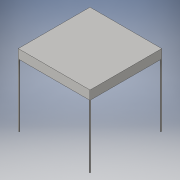
# Autodesk Inventor part: Pit
Saved by Autodesk Inventor 2016 SP2 (Build 200236200, 236)
## iProperties
Created: 2018-01-20
Part Number: Pit
Material: Generic
Document SubType Name: Modeling
Designer: CAD
Density: 1 g/cm^3
Appearance: Default
Author: CAD
Autodesk Inventor part; units mm, degrees
ref_plane "YZ Plane" through (0, 0, 0) normal (1, 0, 0) x (0, 1, 0)
ref_plane "XZ Plane" through (0, 0, 0) normal (0, 1, 0) x (-1, 0, 0)
ref_plane "XY Plane" through (0, 0, 0) normal (0, 0, 1) x (1, 0, 0)
sketch "Sketch1" plane through (0, 0, 0) normal (0, 0, 1) x (1, 0, 0)
  line L0 (0, 0) -> (0, 2438.4)
  line L1 (0, 2438.4) -> (2438.4, 2438.4)
  line L2 (2409.825, 2133.6) -> (28.575, 2133.6)
  line L3 (2438.4, 2438.4) -> (2438.4, 0)
  line L4 (2409.825, 0) -> (2409.825, 2133.6)
  line L5 (28.575, 2133.6) -> (28.575, 0)
  line L6 (0, 0) -> (28.575, 0)
  line L7 (2409.825, 0) -> (2438.4, 0)
  dimension "d0" = 0
  dimension "d1" = 2438.4
  dimension "d3" = 2438.4
  dimension "d4" = 304.8
  dimension "d5" = 28.575
  dimension "d7" = 28.575
  constraints: 16 end point, 2 horizontal, 1 collinear, 1 parallel, 1 vertical
  measures "d0" horizontal distance of L0.start L0.end
  measures "d1" distance of L0.start L0.end
  measures "d3" distance of L0.end L1.end
  measures "d4" distance between parallel lines of L1 L2
  measures "d5" distance between parallel lines of L3 L4
  measures "d7" distance between parallel lines of L0 L5
extrude "Extrusion1" add sketch "Sketch1" along normal blind 2438.4
sketch "Sketch2" plane through (2438.4, 0, 0) normal (1, 0, 0) x (0, 0, -1)
  line L0 (0, 2438.4) -> (-2438.4, 2438.4) projected
  line L1 (-2438.4, 0) -> (-2438.4, 2438.4) projected
  line L2 (0, 2438.4) -> (0, 0) projected
  line L3 (-2409.825, 0) -> (-2409.825, 2133.6)
  line L4 (-28.575, 2133.6) -> (-28.575, 0)
  line L5 (-2409.825, 2133.6) -> (-28.575, 2133.6)
  line L6 (0, 0) -> (-2438.4, 0) projected
  line L7 (-2409.825, 0) -> (-28.575, 0)
  dimension "d10" = 28.575
  dimension "d11" = 28.575
  dimension "d12" = 2133.6
  dimension "d13" = 2133.6
  dimension "d14" = 304.8
  constraints: 8 end point, 1 horizontal
  measures "d10" distance between parallel lines of L1 L3
  measures "d11" distance between parallel lines of L2 L4
  measures "d12" distance of L3.start L3.end
  measures "d13" distance of L4.start L4.end
  measures "d14" distance between parallel lines of L5 L0
extrude "Extrusion2" cut sketch "Sketch2" against normal blind 2438.4 contours L6 L3 L5 L4
sketch "Sketch3" plane through (28.575, 2133.6, 0) normal (0, -1, 0) x (1, 0, 0)
  line L0 (2381.25, 2409.825) -> (2381.25, 2438.4) projected
  line L1 (0, 2409.825) -> (0, 2438.4) projected
  line L2 (2381.25, 2409.825) -> (0, 2409.825)
  line L3 (0, 28.575) -> (-28.575, 28.575) projected
  line L4 (0, 2409.825) -> (0, 28.575)
  line L5 (0, 28.575) -> (2381.25, 28.575)
  line L6 (2381.25, 28.575) -> (2381.25, 2409.825)
  point P0 (-28.575, 0)
  constraints: 8 end point, 3 perpendicular, 1 horizontal
extrude "Extrusion3" cut sketch "Sketch3" against normal blind 276.225
sketch "Sketch4" plane through (28.575, 2133.6, 28.575) normal (0, 0, 1) x (1, 0, 0)
  line L0 (2381.25, 0) -> (2381.25, 276.225) projected
  line L1 (2381.25, 276.225) -> (0, 276.225) projected
  line L2 (0, 0) -> (0, 276.225) projected
  line L3 (-28.575, 304.8) -> (2409.825, 304.8) projected
  line L4 (0, 276.225) -> (2381.25, 276.225) projected
  line L5 (1190.625, 276.225) -> (1190.625, 0)
  line L6 (0, 276.225) -> (550.3563, 148.5423)
  line L7 (595.3125, 138.1125) -> (1190.625, 0)
  line L8 (0, 20.8597) -> (550.3563, 148.5423)
  line L9 (595.3125, 158.9722) -> (1100.7126, 276.225)
  line L10 (89.9124, 276.225) -> (595.3125, 158.9722)
  line L11 (640.2687, 148.5423) -> (1190.625, 20.8597)
  line L12 (0, 0) -> (595.3125, 138.1125)
  line L13 (640.2687, 148.5423) -> (1190.625, 276.225)
  line L14 (2381.25, 0) -> (1785.9375, 138.1125)
  line L15 (1740.9813, 148.5423) -> (1190.625, 276.225)
  line L16 (2291.3376, 276.225) -> (1785.9375, 158.9722)
  line L17 (1740.9813, 148.5423) -> (1190.625, 20.8597)
  line L18 (2381.25, 20.8597) -> (1830.8937, 148.5423)
  line L19 (1785.9375, 158.9722) -> (1280.5374, 276.225)
  line L20 (2381.25, 276.225) -> (1830.8937, 148.5423)
  line L21 (1785.9375, 138.1125) -> (1190.625, 0)
  point P0 (-28.575, -2133.6)
  point P1 (2385.8423, 19.7943)
  point P2 (1195.2173, 296.0193)
  point P3 (2376.6577, 296.0193)
  point P4 (-4.5923, 19.7943)
  point P5 (1186.0327, 296.0193)
  point P6 (4.5923, 296.0193)
  dimension "d26" = 606.4093
  dimension "d29" = 518.8231
  dimension "d31" = 564.9734
  dimension "d34" = 611.1236
  dimension "d35" = 611.1236
  dimension "d36" = 569.6876
  dimension "d37" = 564.9734
  dimension "d38" = 564.9734
  dimension "d39" = 89.9124
  dimension "d40" = 1010.8001
  dimension "d41" = 1010.8001
  dimension "d42" = 564.9734
  dimension "d43" = 564.9734
  constraints: 34 end point, 7 equal length, 7 point on line, 4 parallel, 3 symmetric about line, 1 midpoint, 1 perpendicular
  measures "d26" distance of point (4.592, 296.019) L9.start
  measures "d29" distance of L9.start L9.end
  measures "d31" distance of L11.start L5.start
  measures "d34" distance of L7.start L5.end
  measures "d35" distance of L2.start L7.start
  measures "d36" distance of point (-4.592, 19.794) L6.end
  measures "d37" distance of L1.end L6.end
  measures "d38" distance of L11.start L11.end
  measures "d39" distance of L11.start L6.end
  measures "d40" distance of L9.end L10.start
  measures "d41" distance of L16.start L19.end
  measures "d42" distance of L8.start L6.end
  measures "d43" distance of L18.start L18.end
extrude "Extrusion4" add sketch "Sketch4" along normal blind 20.32 contours L14 L21 L5 L17 L15 L1 L19 L16 L20 L18 L0 | L7 L12 L2 L8 L6 L1 L10 L9 L13 L11 L5
sketch "Sketch6" plane through (28.575, 2133.6, 2409.825) normal (1, 0, 0) x (0, 0, -1)
  line L0 (2360.93, 276.225) -> (0, 276.225) projected
  line L1 (1180.465, 276.225) -> (1180.465, 0)
  line L2 (2381.25, 276.225) -> (2360.93, 276.225) projected
  line L3 (2381.25, 276.225) -> (2381.25, 0)
  line L4 (1180.465, 276.225) -> (1717.1258, 152.7732)
  line L5 (1780.8575, 138.1125) -> (2381.25, 0)
  line L6 (2253.7866, 276.225) -> (1780.8575, 167.4338)
  line L7 (1717.1258, 152.7732) -> (1180.465, 29.3213)
  line L8 (2381.25, 29.3213) -> (1844.5892, 152.7732)
  line L9 (1780.8575, 167.4338) -> (1307.9284, 276.225)
  line L10 (1180.465, 0) -> (1780.8575, 138.1125)
  line L11 (1844.5892, 152.7732) -> (2381.25, 276.225)
  line L12 (-20.32, 29.3213) -> (-20.32, 0)
  line L13 (1180.465, 276.225) -> (643.8042, 152.7732)
  line L14 (580.0725, 138.1125) -> (0, 4.6744)
  line L15 (107.1434, 276.225) -> (580.0725, 167.4338)
  line L16 (643.8042, 152.7732) -> (1180.465, 29.3213)
  line L17 (0, 33.9957) -> (516.3408, 152.7732)
  line L18 (580.0725, 167.4338) -> (1053.0016, 276.225)
  line L19 (1180.465, 0) -> (580.0725, 138.1125)
  line L20 (516.3408, 152.7732) -> (0, 276.225)
  line L21 (0, 33.9957) -> (0, 4.6744)
  line L22 (0, 0) -> (0, 276.225) projected
  line L23 (2253.7866, 276.225) -> (2381.25, 276.225)
  line L24 (107.1434, 276.225) -> (0, 276.225)
  line L25 (1053.0016, 276.225) -> (1180.465, 276.225)
  line L26 (2253.7866, 276.225) -> (2381.25, 276.225)
  line L27 (2409.825, 304.8) -> (-28.575, 304.8) projected
  line L28 (2381.25, 0) -> (2360.93, 0) projected
  line L29 (2381.25, 0) -> (2381.25, 29.3213)
  line L30 (2381.25, 20.8597) -> (2381.25, 148.5423) projected
  point P0 (2409.825, -2133.6)
  point P1 (-20.32, 276.225)
  dimension "d68" = 28.575
  dimension "d69" = 28.575
  dimension "d70" = 28.575
  dimension "d71" = 28.575
  dimension "d73" = 616.0732
  dimension "d75" = 485.2808
  dimension "d76" = 485.2808
  dimension "d77" = 25.91
  dimension "d79" = 276.225
  dimension "d80" = 167.045
  dimension "d81" = 167.045
  dimension "d82" = 20.32
  dimension "d83" = 276.225
  constraints: 50 end point, 8 point on line, 7 symmetric about line, 3 parallel, 2 perpendicular, 1 collinear, 1 midpoint
  measures "d68" distance between parallel lines of L9 L4
  measures "d69" distance between parallel lines of L5 L8
  measures "d70" distance between parallel lines of L6 L11
  measures "d71" distance between parallel lines of L10 L7
  measures "d73" distance of L1.end L5.start
  measures "d75" distance of L6.end L9.end
  measures "d76" distance of L6.start L6.end
  measures "d77" angle of L11 L8
  measures "d79" distance of L1.start L1.end
  measures "d80" angle of L2 L14
  measures "d81" angle of L2 L17
  measures "d82" distance between parallel lines of L12 L22
  measures "d83" distance from line of L12.end L0
extrude "Extrusion5" add sketch "Sketch6" along normal blind 20.32 contours L2 L11 L8 L3 L5 L10 L1 L7 L4 L0 L9 L6 | L13 L16 L1 L19 L14 L21 L17 L20 L0 L15 L18
sketch "Sketch7" plane through (2409.825, 2133.6, 2409.825) normal (0, 0, -1) x (-1, 0, 0)
  line L0 (0, 276.225) -> (550.3563, 148.5423) projected
  line L1 (550.3563, 148.5423) -> (0, 20.8597) projected
  line L2 (595.3125, 138.1125) -> (1190.625, 0) projected
  line L3 (1100.7126, 276.225) -> (595.3125, 158.9722) projected
  line L4 (640.2687, 148.5423) -> (1190.625, 276.225) projected
  line L5 (1190.625, 20.8597) -> (640.2687, 148.5423) projected
  line L6 (0, 0) -> (595.3125, 138.1125) projected
  line L7 (595.3125, 158.9722) -> (89.9124, 276.225) projected
  line L8 (2409.825, 304.8) -> (-28.575, 304.8) projected
  line L9 (1190.625, 0) -> (1785.9375, 138.1125) projected
  line L10 (1190.625, 276.225) -> (1740.9813, 148.5423) projected
  line L11 (1785.9375, 158.9722) -> (1280.5374, 276.225) projected
  line L12 (1740.9813, 148.5423) -> (1190.625, 20.8597) projected
  line L13 (1785.9375, 138.1125) -> (2360.93, 4.7142) projected
  line L14 (2360.93, 25.5739) -> (1830.8937, 148.5423) projected
  line L15 (2291.3376, 276.225) -> (1785.9375, 158.9722) projected
  line L16 (2381.25, 276.225) -> (2360.93, 276.225) projected
  line L17 (1830.8937, 148.5423) -> (2381.25, 276.225)
  line L18 (0, 276.225) -> (89.9124, 276.225)
  line L19 (0, 0) -> (0, 20.8597)
  line L20 (2291.3376, 276.225) -> (2381.25, 276.225)
  line L21 (1100.7126, 276.225) -> (1280.5374, 276.225)
  line L22 (0, 0) -> (0, 20.8597)
  line L23 (595.3125, 138.1125) -> (0, 0)
  line L24 (0, 20.8597) -> (550.3563, 148.5423)
  line L25 (0, 276.225) -> (550.3563, 148.5423)
  line L26 (595.3125, 158.9722) -> (89.9124, 276.225)
  line L27 (595.3125, 158.9722) -> (1100.7126, 276.225)
  line L28 (1190.625, 276.225) -> (640.2687, 148.5423)
  line L29 (640.2687, 148.5423) -> (1190.625, 20.8597)
  line L30 (1190.625, 0) -> (595.3125, 138.1125)
  line L31 (1190.625, 0) -> (1785.9375, 138.1125)
  line L32 (1190.625, 20.8597) -> (1740.9813, 148.5423)
  line L33 (1190.625, 276.225) -> (1740.9813, 148.5423)
  line L34 (1785.9375, 158.9722) -> (1280.5374, 276.225)
  line L35 (1785.9375, 158.9722) -> (2291.3376, 276.225)
  line L36 (1830.8937, 148.5423) -> (2360.93, 25.5739)
  line L37 (2360.93, 4.6744) -> (2360.93, 25.5739)
  line L38 (2360.93, 4.6744) -> (1785.9375, 138.1125)
  point P0 (2361.1019, 271.5506)
  point P1 (2381.25, 0)
  dimension "d88" = 13.062
  dimension "d89" = 166.6875
  constraints: 44 end point, 10 collinear, 4 parallel, 1 perpendicular
  measures "d88" angle of L8 L30
  measures "d89" distance from line of L30.end L8
extrude "Extrusion6" add sketch "Sketch7" along normal blind 20.32
sketch "Sketch8" plane through (2409.825, 2154.4597, 28.575) normal (-1, 0, 0) x (0, 0, 1)
  line L0 (20.32, -16.1853) -> (600.3925, 117.2528) projected
  line L1 (536.6608, 131.9135) -> (0, 8.4616) projected
  line L2 (0, 255.3653) -> (536.6608, 131.9135) projected
  line L3 (600.3925, 146.5741) -> (127.4634, 255.3653) projected
  line L4 (1073.3216, 255.3653) -> (600.3925, 146.5741) projected
  line L5 (1200.785, 8.4616) -> (664.1242, 131.9135) projected
  line L6 (664.1242, 131.9135) -> (1200.785, 255.3653) projected
  line L7 (600.3925, 117.2528) -> (1200.785, -20.8597) projected
  line L8 (1737.4458, 131.9135) -> (1200.785, 8.4616) projected
  line L9 (1200.785, -20.8597) -> (1801.1775, 117.2528) projected
  line L10 (1200.785, 255.3653) -> (1737.4458, 131.9135) projected
  line L11 (1801.1775, 146.5741) -> (1328.2484, 255.3653) projected
  line L12 (1864.9092, 131.9135) -> (2381.25, 255.3653) projected
  line L13 (2381.25, -2154.4597) -> (2409.825, -2154.4597) projected
  line L14 (-28.575, 283.9403) -> (2409.825, 283.9403) projected
  line L15 (-28.575, -2154.4597) -> (0, -2154.4597) projected
  line L16 (2274.1066, 255.3653) -> (1801.1775, 146.5741) projected
  line L17 (2381.25, 13.136) -> (1864.9092, 131.9135) projected
  line L18 (1801.1775, 117.2528) -> (2381.25, -16.1853) projected
  line L19 (2360.93, 255.3653) -> (20.32, 255.3653) projected
  line L20 (0, 0) -> (0, 255.3653) projected
  line L21 (0, 0) -> (20.32, 0) projected
  line L22 (20.32, 0) -> (20.32, -20.8597) projected
  line L23 (2360.93, -20.8597) -> (2360.93, 0) projected
  line L24 (2360.93, 0) -> (2381.25, 0) projected
  line L25 (2381.25, 0) -> (2381.25, 255.3653) projected
  line L26 (2381.25, 255.3653) -> (2360.93, 255.3653) projected
  line L27 (0, 255.3653) -> (536.6608, 131.9135)
  line L28 (536.6608, 131.9135) -> (0, 8.4616)
  line L29 (127.4634, 255.3653) -> (600.3925, 146.5741)
  line L30 (20.32, -16.1853) -> (600.3925, 117.2528)
  line L31 (600.3925, 117.2528) -> (1200.785, -20.8597)
  line L32 (1200.785, 8.4616) -> (664.1242, 131.9135)
  line L33 (664.1242, 131.9135) -> (1200.785, 255.3653)
  line L34 (600.3925, 146.5741) -> (1073.3216, 255.3653)
  line L35 (1200.785, -20.8597) -> (1801.1775, 117.2528)
  line L36 (1737.4458, 131.9135) -> (1200.785, 8.4616)
  line L37 (1200.785, 255.3653) -> (1737.4458, 131.9135)
  line L38 (1328.2484, 255.3653) -> (1801.1775, 146.5741)
  line L39 (1801.1775, 117.2528) -> (2360.93, -11.511)
  line L40 (1864.9092, 131.9135) -> (2381.25, 13.136)
  line L41 (1864.9092, 131.9135) -> (2381.25, 255.3653)
  line L42 (1801.1775, 146.5741) -> (2274.1066, 255.3653)
  line L43 (2274.1066, 255.3653) -> (2381.25, 255.3653)
  line L44 (2360.93, -20.8597) -> (20.32, -20.8597) projected
  line L45 (2360.93, -11.511) -> (2360.93, 0)
  line L46 (2360.93, 127.6827) -> (2360.93, 0) projected
  line L47 (2360.93, 0) -> (2381.25, 13.136)
  line L48 (20.32, -16.1853) -> (20.32, 0)
  line L49 (20.32, 0) -> (0, 8.4616)
  line L50 (20.32, 255.3653) -> (0, 255.3653) projected
  line L51 (0, 255.3653) -> (127.4634, 255.3653)
  constraints: 44 end point, 10 collinear, 5 parallel, 2 point on line
extrude "Extrusion7" add sketch "Sketch8" along normal blind 20.32 contours L22 L49 L1 L2 L50 L19 L3 L4 L11 L16 L26 L12 L17 L46 L23 L18 L9 L7 L0 | L46 L17 L47
body "Solid1"
